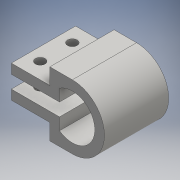
# Autodesk Inventor part: DShaftClamp
Saved by Autodesk Inventor 2016 (Build 200138000, 138)
## iProperties
Created: 2017-11-27
Part Number: DShaftClamp
Material: Generic
Document SubType Name: Modeling
Designer: alex
Density: 1 g/cm^3
Appearance: Default
Author: alex
Autodesk Inventor part; units mm, degrees
ref_plane "YZ Plane" through (0, 0, 0) normal (1, 0, 0) x (0, 1, 0)
ref_plane "XZ Plane" through (0, 0, 0) normal (0, 1, 0) x (-1, 0, 0)
ref_plane "XY Plane" through (0, 0, 0) normal (0, 0, 1) x (1, 0, 0)
sketch "Sketch1" plane through (0, 0, 0) normal (0, 1, 0) x (-1, 0, 0)
  arc A0 (0, 10) -> (0, -10) centre (0, 0) ccw
  line L0 (7, 10) -> (0, 10)
  line L1 (0, 10) -> (0, -10)
  line L2 (0, -10) -> (7, -10)
  line L3 (19, 2) -> (7, 2)
  line L4 (7, -2) -> (19, -2)
  arc A1 (4, 5.7446) -> (4, -5.7446) centre (0, 0) ccw
  line L5 (19, -5) -> (19, -2)
  line L6 (19, 2) -> (19, 5)
  line L7 (6.8374, 10) -> (3.8374, 10)
  line L8 (3.8374, -10) -> (6.8374, -10)
  line L9 (7, 2) -> (4, 2)
  line L10 (7, -2) -> (4, -2)
  line L11 (4, 5.7446) -> (4, 2)
  line L12 (4, -2) -> (4, -5.7446)
  line L13 (7, 10) -> (7, 5)
  line L14 (7, 5) -> (19, 5)
  line L15 (7, -10) -> (7, -5)
  line L16 (7, -5) -> (19, -5)
  point P0 (15, 0)
  point P1 (15, 0)
  dimension "d0" = 20
  dimension "d2" = 3
  dimension "d40" = 3
  dimension "d41" = 3
  dimension "d70" = 4
  dimension "d71" = 4
  dimension "d72" = 15
  dimension "d73" = 15
  dimension "d74" = 12
  dimension "d75" = 4
  dimension "d103" = 5
  dimension "d112" = 4
  dimension "d113" = 12
  dimension "d114" = 12
  dimension "d115" = 12
  dimension "d116" = 12.1626
  dimension "d117" = 12.1626
  dimension "d118" = 15.1626
  dimension "d119" = 15.1626
  constraints: 34 end point, 8 parallel, 7 perpendicular, 6 coincident, 4 point on circle, 3 horizontal, 3 tangent, 2 centre point, 1 horizontal alignment, 1 midpoint
  measures "d0" diameter of A0
  measures "d2" radial gap between concentric circles of A0 A1
  measures "d40" distance of L3.start L6.end
  measures "d41" distance of L5.start L4.end
  measures "d70" distance from line of A1.centre L12
  measures "d71" distance between parallel lines of L1 L11
  measures "d72" distance between parallel lines of L11 L6
  measures "d73" distance between parallel lines of L12 L5
  measures "d74" distance between parallel lines of L13 L6
  measures "d75" distance between parallel lines of L3 L4
  measures "d103" distance between parallel lines of L2 L16
  measures "d112" distance from line of point (15, 0) L5
  measures "d113" distance between parallel lines of L8 L3
  measures "d114" distance from line of L3.end L6
  measures "d115" distance from line of L4.start L6
  measures "d116" distance from line of L7.start L6
  measures "d117" distance from line of L8.end L6
  measures "d118" distance from line of L7.end L6
  measures "d119" distance from line of L8.start L6
extrude "Extrusion1" add sketch "Sketch1" along normal blind 20 contours L1 A1 A0 | L0 L13 L14 L6 L3 L9 L11 A1 L1 | L1 A1 L12 L10 L4 L5 L16 L15 L2
sketch "Sketch2" plane through (-19, 0, 5) normal (0, 0, 1) x (1, 0, 0)
  circle A0 centre (4, 5) radius 1.5
  circle A1 centre (4, 15) radius 1.5
  line L0 (0, 20) -> (12, 20) projected
  line L1 (0, 0) -> (12, 0) projected
  line L2 (0, 0) -> (0, 20) projected
  point P0 (19, 0)
  dimension "d120" = 3
  dimension "d121" = 5
  dimension "d122" = 5
  dimension "d123" = 4
  dimension "d124" = 3
  constraints: 2 centre point, 1 vertical alignment
  measures "d120" diameter of A0
  measures "d121" distance from line of L0 A1.centre
  measures "d122" distance from line of L1 A0.centre
  measures "d123" distance from line of L2 A0.centre
  measures "d124" diameter of A1
extrude "Extrusion2" cut sketch "Sketch2" against normal through all
body "Solid1"
